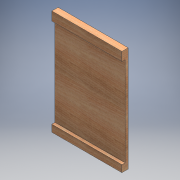
# Autodesk Inventor part: tablero_chico
Saved by Autodesk Inventor 2016 (Build 200138000, 138)
## iProperties
Created: 2018-06-24
Part Number: tablero_chico
Material: Wood (Birch)
Document SubType Name: Modeling
Designer: damia
Density: 0.55 g/cm^3
Appearance: Birch - Natural Polished
Mass: 2732.4 g
Surface Area: 5480.4 cm^2
Volume: 4968 cm^3
Author: damia
Autodesk Inventor part; units mm, degrees
ref_plane "YZ Plane" through (0, 0, 0) normal (1, 0, 0) x (0, 1, 0)
ref_plane "XZ Plane" through (0, 0, 0) normal (0, 1, 0) x (-1, 0, 0)
ref_plane "XY Plane" through (0, 0, 0) normal (0, 0, 1) x (1, 0, 0)
sketch "Sketch2" plane through (0, 0, 0) normal (0, 1, 0) x (-1, 0, 0)
  line L0 (0, 0) -> (-800, 0)
  line L1 (-800, 0) -> (-800, -600)
  line L2 (-800, -600) -> (0, -600)
  line L3 (0, -600) -> (0, 0)
  dimension "d4" = 800
  dimension "d5" = 600
  constraints: 8 end point, 2 parallel, 1 horizontal, 1 perpendicular
  measures "d4" distance of L2.end L1.end
  measures "d5" distance of L1.end L0.end
extrude "Extrusion2" add sketch "Sketch2" along normal blind 18
sketch "Sketch3" plane through (0, 0, 0) normal (0, -1, 0) x (1, 0, 0)
  line L0 (0, -600) -> (0, 0) projected
  line L1 (800, 0) -> (800, -600) projected
  line L2 (0, 0) -> (800, 0)
  line L3 (800, 0) -> (800, -50)
  line L4 (800, -50) -> (0, -50)
  line L5 (0, -50) -> (0, 0)
  dimension "d8" = 50
  constraints: 8 end point, 2 parallel, 1 horizontal, 1 perpendicular, 1 point on line
  measures "d8" distance of L2.end L3.end
extrude "Extrusion3" add sketch "Sketch3" along normal blind 18
sketch "Sketch4" plane through (0, 0, 0) normal (0, -1, 0) x (1, 0, 0)
  line L0 (0, -600) -> (0, 0) projected
  line L1 (800, 0) -> (800, -600) projected
  line L2 (0, -600) -> (800, -600)
  line L3 (800, -600) -> (800, -560)
  line L4 (800, -560) -> (0, -560)
  line L5 (0, -560) -> (0, -600)
  dimension "d11" = 40
  constraints: 8 end point, 2 parallel, 1 horizontal, 1 perpendicular, 1 point on line
  measures "d11" distance of L3.end L2.end
extrude "Extrusion4" add sketch "Sketch4" along normal blind 18
equation "\"d5\" = Profundidad"
equation "\"Profundidad\" = 600"
body "Solid2"
